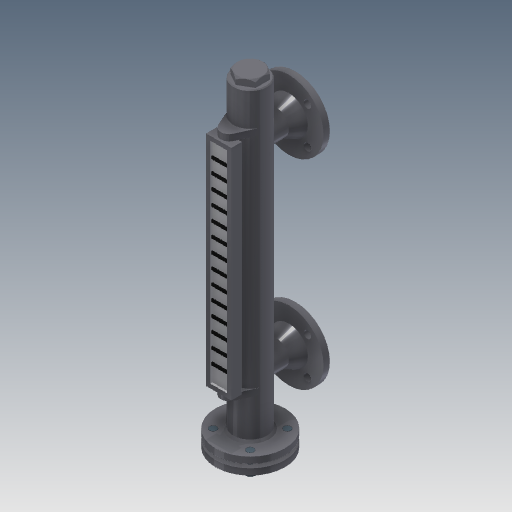
# Autodesk Inventor part: Bypass Level Gauge
Saved by Autodesk Inventor 2020 (Build 240152000, 152)
## iProperties
Shininess: 41.0
Angle Display Precision: 2
Document Length Units: 11269
Document Angle Units: 11279
Document Time Units: 11290
Document Mass Units: 11283
Document Length Units Precision: 3
Document Angle Units Precision: 2
NAME: PIPING: BS4504 Flange PN16
DATA: <meta><inlinegroups number="0" deflen="0"></inlinegroups><connections number="1"></connections><angles></angles></meta>
Created: 2002-04-25
Part Number: Bypass Level Gauge
Material: Cast Iron
Document SubType Name: Modeling
Designer: D.Ali
Description: Vessel Level Gauge
Standard: BS4504
Standard Revision: 1
Manufacturer: Datech
Standards Organization: Custom
Language: ENG
Categories: <domain><piping version="1" type="fitting"><fitting><connection index="1" flipDirection="False"><display>Connection1</display><NS><bound-to>ND</bound-to></NS><Female>False</Female><EndTreatment>Flanged</EndTreatment><Fixed>False</Fixed><MaxEngagement> 0</MaxEngagement><MinEngagement> 0</MinEngagement></connection></fitting></piping></domain>
Density: 7.05 g/cm^3
Appearance: Metal-Steel (Polished)
Stock Number: NA
Mass: 41827.6 g
Surface Area: 5425.44 cm^2
Volume: 5932.99 cm^3
Density: 0.0
Volumn: 0.0
Area: 0.0
PropertySet Name: Model Information
Control State: 0
Master: False
Checked Out: False
Face_face: 229.000 mm
NB: 100.000 mm
PCD: 180.000 mm
FlangeOD: 220.000 mm
Holenum: 8.000 ul
FlangefaceOD: 156.000 mm
Holedia: 19.000 mm
Flangethk: 16.000 mm
PipeOD: 110.000 mm
Flangefacethk: 3.000 mm
Author: Demir Ali
Title: Purchased Part
Revision Number: A
Autodesk Inventor part; units mm, degrees
ref_plane "YZ Plane" through (0, 0, 0) normal (1, 0, 0) x (0, 1, 0)
ref_plane "XZ Plane" through (0, 0, 0) normal (0, 1, 0) x (-1, 0, 0)
ref_plane "XY Plane" through (0, 0, 0) normal (0, 0, 1) x (1, 0, 0)
sketch "Sketch27" plane through (0, 0, 0) normal (0, 1, 0) x (-1, 0, 0)
  circle A0 centre (0, 0) radius 82.5
  dimension "d21" = 165
  constraints: 1 centre point, 1 coincident
  measures "d21" diameter of A0
extrude "Extrusion20" add sketch "Sketch27" against normal blind 15
sketch "Sketch55" plane through (0, -15, 0) normal (0, -1, 0) x (1, 0, 0)
  circle A0 centre (0, 0) radius 82.5 projected
  circle A1 centre (0, 0) radius 51
  dimension "d275" = 102
  constraints: 1 centre point, 1 coincident
  measures "d275" diameter of A1
extrude "Extrusion39" add sketch "Sketch55" along normal blind 3 contours A1
chamfer "Chamfer8" distance 3 angle 45 1 edges at (-51, -15, 0)
sketch "Sketch29" plane through (0, 0, 0) normal (0, 1, 0) x (1, 0, 0)
  circle A0 centre (0, 0) radius 62.5
  circle A1 centre (0, 0) radius 62.5 construction
  line L0 (0, 0) -> (-44.1942, -44.1942) construction
  circle A2 centre (0, 0) radius 82.5 projected
  line L1 (0, 115.5) -> (0, -115.5) projected
  dimension "d29" = 125
  dimension "d30" = 45
  constraints: 3 coincident, 2 end point, 6 other
  measures "d30" angle of L1 L0
hole "Hole2" at (-44.1942, 0, 44.1942) direction (0, -1, 0) diameter 18 end through all
pattern_circular "Circular Pattern2" count 4 over 360 about axis through (0, 0, 0) along (0, -1, 0) of "Hole2"
sketch "Sketch57" plane through (0, -18, 0) normal (0, -1, 0) x (1, 0, 0)
  circle A0 centre (0, 0) radius 51 projected
  circle A1 centre (0, 0) radius 30.1625
  dimension "d288" = 60.325
  constraints: 1 centre point
  measures "d288" diameter of A1
extrude "Extrusion40" add sketch "Sketch57" against normal blind 109.982 contours A1
chamfer "Chamfer9" distance 15 distance2 30 1 edges at (-30.1625, 0, 0) measured on face at (-30.6625, 0, 0)
sketch "Sketch58" plane through (0, 0, 0) normal (0, 0, 1) x (1, 0, 0)
  line L0 (-30.1625, 91.982) -> (30.1625, 91.982) projected
  circle A0 centre (0, 91.982) radius 40
  dimension "d294" = 80
  constraints: 1 centre point, 1 midpoint
  measures "d294" diameter of A0
sketch "Sketch71" plane through (0, -18, 0) normal (0, -1, 0) x (1, 0, 0)
  circle A0 centre (0, 0) radius 51 projected
  circle A1 centre (0, 0) radius 25
  dimension "d390" = 50
  constraints: 1 centre point
  measures "d390" diameter of A1
extrude "Extrusion53" cut sketch "Sketch71" against normal through all contours A1
extrude "Extrusion41" add sketch "Sketch58" along normal blind 125
pattern_linear "Connection2" count 2 spacing 475 along (0, 0, -1) of "Extrusion20", "Extrusion39", "Chamfer8", "Hole2", "Circular Pattern2", "Extrusion40", "Chamfer9", "Extrusion53"
extrude "Extrusion42" add sketch "Sketch58" against normal blind 600
ref_plane "Midplane" through (0, 91.982, -237.5) normal (0, 0, 1) x (1, 0, 0)
sketch "Sketch59" plane through (0, 91.982, 125) normal (0, 0, 1) x (1, 0, 0)
  line L0 (0, 34.641) -> (30, 17.3205)
  line L1 (30, 17.3205) -> (30, -17.3205)
  line L2 (30, -17.3205) -> (0, -34.641)
  line L3 (0, -34.641) -> (-30, -17.3205)
  line L4 (-30, -17.3205) -> (-30, 17.3205)
  line L5 (-30, 17.3205) -> (0, 34.641)
  circle A0 centre (0, 0) radius 40 projected
  point P0 (0, 0)
  point P1 (0, 0)
  dimension "d302" = 60
  dimension "d308" = 69.282
  constraints: 12 end point, 2 coincident, 1 vertical, 11 other
  measures "d302" distance between parallel lines of L4 L1
  measures "d308" distance of L2.end L0.start
extrude "Extrusion43" add sketch "Sketch59" along normal blind 16 contours L0 L1 L2 L3 L4 L5
sketch "Sketch60" plane through (0, 0, 0) normal (1, 0, 0) x (0, 1, 0)
  line L0 (57.341, 141) -> (57.341, 136)
  line L1 (57.341, 136) -> (62.341, 141)
  line L2 (0, -602.2) -> (0, 828.6) projected
  line L3 (57.341, 141) -> (62.341, 141)
  line L4 (91.982, -748.2) -> (91.982, 289.2) projected
  dimension "d309" = 5
  dimension "d310" = 5
  constraints: 6 end point, 2 perpendicular
  measures "d309" horizontal distance of L0.end L1.end
  measures "d310" distance of L0.start L1.end
revolve "Revolution1" cut sketch "Sketch60" angle 360 about axis through (0, 91.982, 0) along (0, 0, 1)
chamfer "Chamfer10" distance 2 angle 45 1 edges at (-40, 91.982, 125)
sketch "Sketch61" plane through (0, 91.982, -600) normal (0, 0, -1) x (-1, 0, 0)
  circle A0 centre (0, 0) radius 82.5
  dimension "d314" = 165
  constraints: 1 centre point, 1 coincident
  measures "d314" diameter of A0
extrude "Extrusion44" add sketch "Sketch61" along normal blind 15
sketch "Sketch62" plane through (0, 91.982, -615) normal (0, 0, -1) x (1, 0, 0)
  circle A0 centre (0, 0) radius 82.5 projected
  circle A1 centre (0, 0) radius 51
  dimension "d318" = 102
  constraints: 1 centre point, 1 coincident
  measures "d318" diameter of A1
extrude "Extrusion45" add sketch "Sketch62" along normal blind 3 contours A1
sketch "Sketch63" plane through (0, 91.982, -600) normal (0, 0, 1) x (1, 0, 0)
  circle A0 centre (0, 0) radius 62.5
  circle A1 centre (0, 0) radius 62.5 construction
  line L0 (0, 0) -> (44.1942, 44.1942) construction
  circle A2 centre (0, 0) radius 82.5 projected
  line L1 (0, 99) -> (0, -132) projected
  point P0 (44.1942, 44.1942)
  dimension "d324" = 125
  dimension "d323" = 45
  constraints: 3 coincident, 2 end point, 6 other
  measures "d323" angle of L1 L0
hole "Hole7" at (44.1942, 136.1762, -600) direction (0, 0, -1) diameter 18 end through all
pattern_circular "Circular Pattern4" count 4 over 360 about axis through (0, 91.982, -600) along (0, 0, -1) of "Hole7"
ref_plane "Flange Mirror" through (0, 91.982, -619.5) normal (0, 0, -1) x (-1, 0, 0)
mirror "Mirror6" about plane through (0, 91.982, -619.5) normal (0, 0, -1) of "Extrusion45", "Hole7", "Circular Pattern4", "Extrusion44"
sketch "Sketch64" plane through (0, 91.982, -639) normal (0, 0, -1) x (-1, 0, 0)
  line L0 (-56.1942, 51.1224) -> (-56.1942, 37.266)
  line L1 (-44.1942, 58.0506) -> (-56.1942, 51.1224)
  line L2 (-32.1942, 51.1224) -> (-44.1942, 58.0506)
  line L3 (-32.1942, 37.266) -> (-32.1942, 51.1224)
  line L4 (-44.1942, 30.3378) -> (-32.1942, 37.266)
  line L5 (-56.1942, 37.266) -> (-44.1942, 30.3378)
  circle A0 centre (-44.1942, 44.1942) radius 12 construction
  circle A1 centre (-44.1942, 44.1942) radius 9 projected
  circle A2 centre (-44.1942, 44.1942) radius 8.25
  dimension "d345" = 24
  dimension "d359" = 16.5
  constraints: 12 end point, 6 tangent, 2 centre point, 2 coincident, 2 equal length, 2 parallel, 2 vertical
  measures "d345" diameter of A0
  measures "d359" diameter of A2
extrude "Extrusion46" add sketch "Sketch64" along normal blind 9.2 contours L1 L2 L3 L4 L5 L0 | A1 | A2
extrude "Extrusion47" add sketch "Sketch64" against normal up to surface (39 mm away) contours A2
ref_plane "Work Plane13" through (44.1942, 150.0326, -639) normal (-1, 0, 0) x (0, 0, -1)
ref_plane "Work Plane14" through (38.1942, 132.7121, -639) normal (-0.5, 0.8660254, 0) x (0.8660254, 0.5, 0)
sketch "Sketch65" plane through (44.1942, 150.0326, -639) normal (-1, 0, 0) x (0, 0, -1)
  line L0 (7.2, 27.7128) -> (9.2, 23.7128)
  line L1 (9.2, 23.7128) -> (9.2, 27.7128)
  line L2 (9.2, 27.7128) -> (7.2, 27.7128)
  line L3 (-942.2323, 13.8564) -> (167.7721, 13.8564) projected
  point P0 (9.2, 27.7128)
  dimension "d354" = 4
  dimension "d355" = 2
  constraints: 6 end point, 2 coincident, 1 perpendicular, 1 vertical
  measures "d354" distance of L0.end L1.end
  measures "d355" distance of L1.end L0.start
revolve "Revolution2" cut sketch "Sketch65" angle 360 about axis through (44.1942, 136.1762, -639) along (0, 0, 1)
pattern_circular "Circular Pattern5" count 4 over 360 about axis through (0, 91.982, -639) along (0, 0, -1) of "Revolution2", "Extrusion46", "Extrusion47"
chamfer "Chamfer11" distance 5 angle 45 1 edges at (-40, 91.982, -600)
ref_plane "Work Plane15" through (0, -18, 30.1625) normal (0, 0, 1) x (1, 0, 0)
sketch "Sketch66" plane through (0, -18, 30.1625) normal (0, 0, 1) x (1, 0, 0)
  circle A0 centre (0, 109.982) radius 40 projected
  line L0 (-36.6606, 125.982) -> (-18.3303, 167.982)
  arc A1 (18.3303, 167.982) -> (-18.3303, 167.982) centre (0, 159.982) ccw
  line L1 (18.3303, 167.982) -> (36.6606, 125.982)
  dimension "d365" = 20
  dimension "d366" = 50
  constraints: 4 end point, 4 point on circle, 4 tangent, 1 centre point, 1 vertical alignment
  measures "d365" radius of A1
  measures "d366" distance of A0.centre A1.centre
extrude "Extrusion48" add sketch "Sketch66" along normal blind 15
pattern_linear "Rectangular Pattern2" count 2 spacing 535.325 along (0, 0, -1) of "Extrusion48"
sketch "Sketch67" plane through (0, 141.982, -490.1625) normal (0, 0, 1) x (1, 0, 0)
  arc A0 (18.3303, 8) -> (-18.3303, 8) centre (0, 0) ccw projected
  line L0 (-30, 25) -> (30, 25)
  line L1 (30, 25) -> (30, 0)
  line L2 (30, 0) -> (-30, 0)
  line L3 (-30, 0) -> (-30, 25)
  point P0 (0, 25)
  dimension "d372" = 25
  dimension "d373" = 60
  constraints: 8 end point, 2 midpoint, 2 parallel, 1 horizontal, 1 perpendicular, 1 vertical alignment
  measures "d372" distance of L0.end L1.end
  measures "d373" distance of L0.start L0.end
extrude "Extrusion49" add sketch "Sketch67" along normal up to surface (520.325 mm away)
sketch "Sketch68" plane through (-30, 166.982, -490.1625) normal (0, 1, 0) x (1, 0, 0)
  line L0 (0, -520.325) -> (60, -520.325) projected
  line L1 (60, 0) -> (60, -520.325) projected
  line L2 (0, 0) -> (60, 0) projected
  line L3 (0, 0) -> (0, -520.325) projected
  line L4 (50, -510.325) -> (10, -510.325)
  line L5 (10, -510.325) -> (10, -10)
  line L6 (10, -10) -> (50, -10)
  line L7 (50, -10) -> (50, -510.325)
  dimension "d376" = 10
  dimension "d384" = 500.325
  constraints: 8 end point, 3 other
  measures "d384" distance of L4.end L5.end
extrude "Extrusion50" cut sketch "Sketch68" against normal blind 5 contours L4 L5 L6 L7
sketch "Sketch70" plane through (-30, 161.982, -490.1625) normal (0, 1, 0) x (1, 0, 0)
  line L0 (50, -510.325) -> (50, -10) projected
  line L1 (50, -10) -> (10, -10) projected
  line L2 (10, -10) -> (10, -510.325) projected
  line L3 (50, -53) -> (10, -53)
  line L4 (10, -53) -> (10, -47)
  line L5 (10, -47) -> (50, -47)
  line L6 (50, -47) -> (50, -53)
  line L7 (50, -50) -> (10, -50) construction
  dimension "d382" = 6
  dimension "d383" = 40
  constraints: 10 end point, 2 midpoint, 2 parallel, 2 point on line, 1 horizontal, 1 perpendicular
  measures "d382" distance between parallel lines of L3 L5
  measures "d383" distance between parallel lines of L7 L1
extrude "Extrusion52" add sketch "Sketch70" along normal blind 3 contours L3 L2 L5 L0
pattern_linear "Rectangular Pattern3" count 14 spacing 32.6883 along (0, 0, 1) of "Extrusion52"
equation "\"NB\" = 50"
equation "\"PipeOD\" = 60.325"
equation "\"FlangeOD\" = 165"
equation "\"FlangefaceOD\" = 102"
equation "\"Holedia\" = 18"
equation "\"Holenum\" = 4"
equation "\"PCD\" = 125"
equation "\"Flangethk\" = 15"
equation "\"Flangefacethk\" = 3"
body "Solid1"
